Autodesk Inventor part; units mm, degrees
(part 2 of 2)
sketch "Skizze7" plane through (0, 0, 46) normal (0, 0, 1) x (1, 0, 0)
  circle A0 centre (-50, 12.5) radius 1.85 projected
  line L0 (-53.4641, 12.5) -> (-51.7321, 15.5)
  line L1 (-51.7321, 15.5) -> (-48.2679, 15.5)
  line L2 (-48.2679, 15.5) -> (-46.5359, 12.5)
  line L3 (-46.5359, 12.5) -> (-48.2679, 9.5)
  line L4 (-48.2679, 9.5) -> (-51.7321, 9.5)
  line L5 (-51.7321, 9.5) -> (-53.4641, 12.5)
  circle A1 centre (-50, 0) radius 1.85 construction
  line L6 (-50, 0) -> (-50, 27) construction
  line L7 (-48, 29) -> (-53, 24) construction
  line L8 (-51.7321, 15.5) -> (-53, 15.5)
  line L9 (-51.7321, 9.5) -> (-53, 9.5)
  line L10 (-53, 24) -> (-53, -24) construction
  line L11 (-53, 0) -> (52.8564, 0) construction
  line L12 (0, 0) -> (0, 29) construction
  line L13 (-53.4641, -12.5) -> (-51.7321, -15.5)
  line L14 (-51.7321, -15.5) -> (-48.2679, -15.5)
  line L15 (-48.2679, -15.5) -> (-46.5359, -12.5)
  line L16 (-46.5359, -12.5) -> (-48.2679, -9.5)
  line L17 (-48.2679, -9.5) -> (-51.7321, -9.5)
  line L18 (-51.7321, -9.5) -> (-53.4641, -12.5)
  line L19 (-51.7321, -15.5) -> (-53, -15.5)
  line L20 (-51.7321, -9.5) -> (-53, -9.5)
  circle A2 centre (50, 12.5) radius 1.85
  line L21 (53.4641, 12.5) -> (51.7321, 15.5)
  line L22 (51.7321, 15.5) -> (48.2679, 15.5)
  line L23 (48.2679, 15.5) -> (46.5359, 12.5)
  line L24 (46.5359, 12.5) -> (48.2679, 9.5)
  line L25 (48.2679, 9.5) -> (51.7321, 9.5)
  line L26 (51.7321, 9.5) -> (53.4641, 12.5)
  line L27 (51.7321, 15.5) -> (53, 15.5)
  line L28 (51.7321, 9.5) -> (53, 9.5)
  line L29 (51.7321, -15.5) -> (53, -15.5)
  line L30 (53.4641, -12.5) -> (51.7321, -15.5)
  line L31 (51.7321, -15.5) -> (48.2679, -15.5)
  line L32 (48.2679, -15.5) -> (46.5359, -12.5)
  line L33 (46.5359, -12.5) -> (48.2679, -9.5)
  line L34 (48.2679, -9.5) -> (51.7321, -9.5)
  line L35 (51.7321, -9.5) -> (53, -9.5)
  line L36 (51.7321, -9.5) -> (53.4641, -12.5)
  line L37 (-53, 24) -> (-48, 29) projected
  line L38 (-53, 24) -> (-53, -24) projected
  line L39 (-48, -29) -> (-53, -24) projected
  line L40 (-48, -29) -> (48, -29) projected
  line L41 (53, -24) -> (48, -29) projected
  line L42 (53, -24) -> (53, 24) projected
  line L43 (48, 29) -> (53, 24) projected
  line L44 (48, 29) -> (-48, 29) projected
  circle A3 centre (50, 12.5) radius 1.85 projected
  circle A4 centre (50, 0) radius 1.85 projected
  circle A5 centre (50, -12.5) radius 1.85 projected
  circle A6 centre (-50, 12.5) radius 1.85 projected
  circle A7 centre (-50, -12.5) radius 1.85 projected
  circle A8 centre (-50, 0) radius 1.85 projected
  line L45 (-47, -26) -> (47, -26) projected
  line L46 (-47, -26) -> (-47, 26) projected
  line L47 (47, 26) -> (-47, 26) projected
  line L48 (47, 26) -> (47, -26) projected
  line L49 (-53.4641, 0) -> (-51.7321, 3)
  line L50 (-51.7321, 3) -> (-48.2679, 3)
  line L51 (-48.2679, 3) -> (-46.5359, 0)
  line L52 (-46.5359, 0) -> (-48.2679, -3)
  line L53 (-48.2679, -3) -> (-51.7321, -3)
  line L54 (-51.7321, -3) -> (-53.4641, 0)
  line L55 (-51.7321, 3) -> (-53, 3)
  line L56 (-51.7321, -3) -> (-53, -3)
  circle A9 centre (50, 0) radius 1.85 construction
  circle A10 centre (50, 0) radius 1.85
  line L57 (53.4641, 0) -> (51.7321, 3)
  line L58 (51.7321, 3) -> (48.2679, 3)
  line L59 (51.7321, -3) -> (53.4641, 0)
  line L60 (51.7321, -3) -> (53, -3)
  line L61 (48.2679, -3) -> (51.7321, -3)
  line L62 (51.7321, 3) -> (53, 3)
  line L63 (48.2679, 3) -> (46.5359, 0)
  line L64 (46.5359, 0) -> (48.2679, -3)
  point P0 (-50, 15.5)
  point P1 (50, 27)
  point P2 (50, 15.5)
  point P3 (53, -9.5)
  point P4 (53, 9.5)
  point P5 (53, 15.5)
  point P6 (-53, -9.5)
  point P7 (-53, 9.5)
  point P8 (47, 13.3038)
  point P9 (47, 11.6962)
  point P10 (47, -11.6962)
  point P11 (47, -13.3038)
  point P12 (-47, -13.3038)
  point P13 (-47, -11.6962)
  point P14 (-47, 11.6962)
  point P15 (-47, 13.3038)
  point P16 (-50, 3)
  point P17 (53, 0)
  point P18 (50, 3)
  point P19 (47, 0.8038)
  point P20 (47, -0.8038)
  point P21 (-47, -0.8038)
  point P22 (-47, 0.8038)
  dimension "d48" = 6
  dimension "d53" = 6
  constraints: 102 end point, 42 symmetric about line, 9 point on line, 4 coincident, 3 centre point, 3 horizontal, 3 midpoint, 2 vertical, 29 other
  measures "d48" distance between parallel lines of L3 L0
  measures "d53" distance between parallel lines of L52 L49
extrude "Extrusion7" cut sketch "Skizze7" against normal blind 10 contours A0 | L38 L8 L0 | L0 L1 L2 L46 L3 L4 L5 L38 | L5 L9 L38 | L55 L49 L38 | L2 L3 L46 | L49 L50 L51 L46 L52 L53 L54 L38 | L51 L52 L46 | L54 L56 L38 | L48 L24 L23 | L23 L22 L21 L42 L26 L25 L24 L48 | L42 L21 L27 | L46 L15 L14 L13 L38 L18 L17 L16 | L16 L15 L46 | L20 L18 L38 | L63 L58 L57 L42 L59 L61 L64 L48 | L48 L64 L63 | L42 L28 L26 | L13 L19 L38 | L48 L32 L33 | L33 L34 L36 L42 L30 L31 L32 L48 | L62 L42 L57 | L59 L42 L60 | L35 L42 L36 | L30 L42 L29 | A4 | A5 | A7 | A8
extrude "Extrusion8" add sketch "Skizze7" against normal blind 7 contours L38 L8 L0 | L0 L1 L2 L46 L3 L4 L5 L38 | L5 L9 L38 | L55 L49 L38 | L49 L50 L51 L46 L52 L53 L54 L38 | L54 L56 L38 | L23 L22 L21 L42 L26 L25 L24 L48 | L42 L21 L27 | L46 L15 L14 L13 L38 L18 L17 L16 | L20 L18 L38 | L63 L58 L57 L42 L59 L61 L64 L48 | L42 L28 L26 | L13 L19 L38 | L33 L34 L36 L42 L30 L31 L32 L48 | L62 L42 L57 | L59 L42 L60 | L35 L42 L36 | L30 L42 L29
sketch "Skizze8" plane through (53, -24, 0) normal (1, 0, 0) x (0, 0, -1)
  line L0 (-3, -2) -> (-3, 50) projected
  line L1 (-3, 50) -> (-3, -2) projected
  line L2 (-3, 7.85) -> (-3, 0.15) projected
  line L3 (-3, 47.85) -> (-3, 40.15) projected
  line L4 (-3, 47.85) -> (-3, 40.15) projected
  line L5 (-3, 7.85) -> (-3, 0.15) projected
  line L6 (-7, 19.5) -> (-3, 19.5)
  line L7 (-3, 19.5) -> (-3, 28.5)
  line L8 (-3, 28.5) -> (-7, 28.5)
  line L9 (-7, 28.5) -> (-7, 19.5)
  line L10 (0, 24) -> (-46, 24) construction
  line L11 (-46, 22.15) -> (-46, 25.85) construction
  point P0 (-7, 24)
  dimension "d54" = 4
  dimension "d55" = 9
  constraints: 10 end point, 2 midpoint, 2 parallel, 2 point on line, 1 horizontal, 1 perpendicular
  measures "d54" distance of L7.end L8.end
  measures "d55" distance of L8.end L6.start
extrude "Extrusion9" cut sketch "Skizze8" against normal through all
equation "\"d18\" = d10"
equation "\"d20\" = d19"
equation "\"d35\" = d34"
